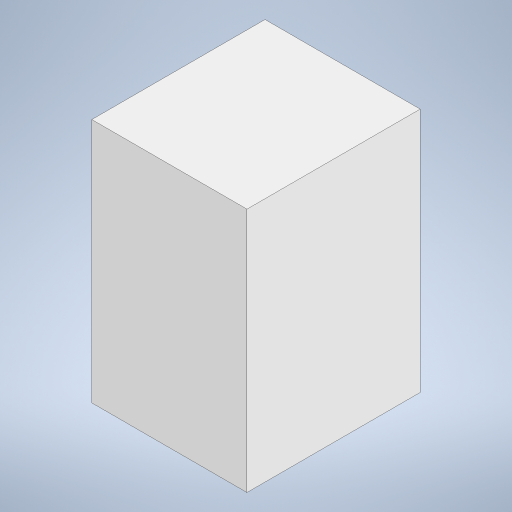
# Autodesk Inventor part: Laundry_Sink
Saved by Autodesk Inventor 2024 (Build 280153000, 153)
## iProperties
Created: 2023-05-15
Part Number: Laundry_Sink
Material: Steel
Document SubType Name: Modeling
Designer: Tom
Density: 7.85 g/cm^3
Appearance: White
Mass: 2.25683e+06 g
Surface Area: 26619.3 cm^2
Volume: 287495 cm^3
Author: Tom
Autodesk Inventor part; units mm, degrees
ref_plane "YZ Plane" through (0, 0, 0) normal (1, 0, 0) x (0, 1, 0)
ref_plane "XZ Plane" through (0, 0, 0) normal (0, 1, 0) x (-1, 0, 0)
ref_plane "XY Plane" through (0, 0, 0) normal (0, 0, 1) x (1, 0, 0)
sketch "Sketch1" plane through (0, 0, 0) normal (1, 0, 0) x (0, 1, 0)
  line L0 (0, 0) -> (863.6, 0)
  line L1 (863.6, 0) -> (863.6, -609.6)
  line L2 (863.6, -609.6) -> (0, -609.6)
  line L3 (0, -609.6) -> (0, 0)
  dimension "d1" = 863.6
  dimension "d2" = 609.6
  constraints: 8 end point, 2 parallel, 1 horizontal, 1 perpendicular
  measures "d1" distance of L1.end L2.end
  measures "d2" distance of L0.end L1.end
extrude "Extrusion1" add sketch "Sketch1" along normal blind 546.1
body "Solid1"
